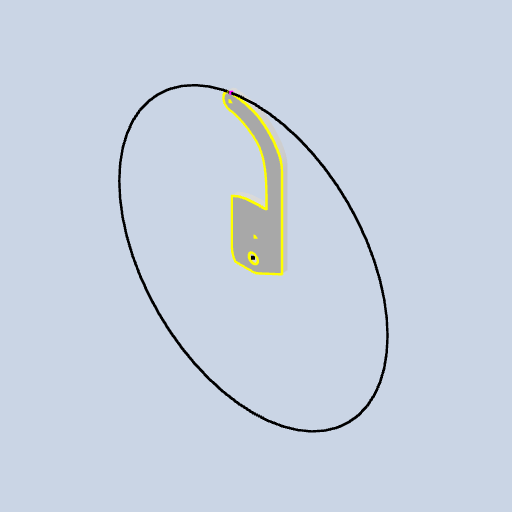
# Autodesk Inventor part: limit_arm
Saved by Autodesk Inventor 2022 (Build 260153000, 153)
## iProperties
Created: 2024-10-15
Part Number: limit_arm
Material: Типовые
Document SubType Name: Modeling
Designer: Andrey
Density: 1 g/cm^3
Appearance: По умолчанию
Author: Andrey
Autodesk Inventor part; units mm, degrees
ref_plane "YZ Plane" through (0, 0, 0) normal (1, 0, 0) x (0, 1, 0)
ref_plane "XZ Plane" through (0, 0, 0) normal (0, 1, 0) x (-1, 0, 0)
ref_plane "XY Plane" through (0, 0, 0) normal (0, 0, 1) x (1, 0, 0)
sketch "Эскиз1" plane through (0, 0, 0) normal (0, 0, 1) x (1, 0, 0)
  line L0 (8.4266, -12.65) -> (-2.5734, -12.65)
  line L1 (-2.5734, -12.65) -> (-2.5734, -47.65)
  line L2 (-2.5734, -47.65) -> (8.4266, -47.65)
  line L3 (8.4266, -47.65) -> (8.4266, -82.9136)
  spline S0 degree 4 poles (2.3773, -93.423) (5.3243, -91.0921) (7.8605, -87.681) (8.4266, -85.6037) (8.4266, -82.9136) knots 0.089011 0.089011 0.089011 0.089011 0.089011 1 1 1 1 1
  spline S1 degree 4 poles (1.3465, -94.1725) (1.6324, -93.9967) (1.8997, -93.813) (2.1479, -93.6217) (2.3773, -93.423) knots 0 0 0 0 0 1 1 1 1 1
  spline S2 degree 4 poles (1.2081, -94.2627) (1.2427, -94.2405) (1.2773, -94.218) (1.3119, -94.1954) (1.3465, -94.1725) knots 0 0 0 0 0 1 1 1 1 1
  spline S3 degree 2 poles (-15.5734, -96.9447) (-3.5967, -97.3511) (1.2081, -94.2627) knots 0 0 0 0.59566 0.59566 0.59566
  line L4 (-125.5734, -96.9447) -> (-15.5734, -96.9447)
  spline S4 degree 2 poles (-125.5734, -96.9447) (-137.55, -97.3511) (-142.3548, -94.2627) knots 0 0 0 0.59566 0.59566 0.59566
  spline S5 degree 4 poles (-142.3548, -94.2627) (-145.6699, -92.132) (-148.8913, -88.0811) (-149.5734, -85.8665) (-149.5734, -82.9136) knots 0 0 0 0 0 1 1 1 1 1
  line L5 (-149.5734, -82.9136) -> (-149.5734, -35.15)
  spline S6 degree 2 poles (-125.5734, 36.6447) (-137.55, 37.0511) (-142.3548, 33.9627) knots 0 0 0 0.59566 0.59566 0.59566
  line L6 (-15.5734, 36.6447) -> (-125.5734, 36.6447)
  spline S7 degree 2 poles (-15.5734, 36.6447) (-3.5967, 37.0511) (1.2081, 33.9627) knots 0 0 0 0.59566 0.59566 0.59566
  spline S8 degree 4 poles (1.2081, 33.9627) (4.5231, 31.832) (7.7445, 27.7811) (8.4266, 25.5665) (8.4266, 22.6136) knots 0 0 0 0 0 1 1 1 1 1
  line L7 (8.4266, 22.6136) -> (8.4266, -12.65)
  line L8 (-10.5734, -92.9447) -> (-10.5734, 32.6447)
  line L9 (-10.5734, 32.6447) -> (-130.5734, 32.6447)
  line L10 (-130.5734, 32.6447) -> (-130.5734, -92.9447)
  line L11 (-130.5734, -92.9447) -> (-10.5734, -92.9447)
  line L12 (5.7794, 10.35) -> (5.7794, -10.35)
  line L13 (-8.4266, 10.35) -> (5.7794, 10.35)
  line L14 (-8.4266, -10.35) -> (-8.4266, 10.35)
  line L15 (5.7794, -10.35) -> (-8.4266, -10.35)
  circle A0 centre (-0.824, -6.35) radius 2.1
  line L16 (-10.5734, 32.6447) -> (-10.5734, -92.9447)
  line L17 (-10.5734, -92.9447) -> (-130.5734, -92.9447)
  line L18 (-130.5734, -92.9447) -> (-130.5734, 32.6447)
  line L19 (-130.5734, 32.6447) -> (-10.5734, 32.6447)
  line L20 (8.4266, -47.65) -> (-2.5734, -47.65)
  line L21 (-2.5734, -47.65) -> (-2.5734, -12.65)
  line L22 (-2.5734, -12.65) -> (8.4266, -12.65)
  line L23 (8.4266, 22.6136) -> (8.4266, -12.65)
  spline S9 degree 4 poles (1.2081, 33.9627) (4.5231, 31.832) (7.7445, 27.7811) (8.4266, 25.5665) (8.4266, 22.6136) knots 0 0 0 0 0 1 1 1 1 1
  spline S10 degree 2 poles (-15.5734, 36.6447) (-3.5967, 37.0511) (1.2081, 33.9627) knots 0 0 0 0.59566 0.59566 0.59566
  line L24 (-125.5734, 36.6447) -> (-15.5734, 36.6447)
  spline S11 degree 2 poles (-142.3548, 33.9627) (-137.55, 37.0511) (-125.5734, 36.6447) knots -0.59566 -0.59566 -0.59566 0 0 0
  spline S12 degree 4 poles (-142.3548, 33.9627) (-145.6699, 31.832) (-148.8913, 27.7811) (-149.5734, 25.5665) (-149.5734, 22.6136) knots 0 0 0 0 0 1 1 1 1 1
  line L25 (-149.5734, 22.6136) -> (-149.5734, -25.15)
  spline S13 degree 2 poles (-125.5734, -96.9447) (-137.55, -97.3511) (-142.3548, -94.2627) knots 0 0 0 0.59566 0.59566 0.59566
  line L26 (-15.5734, -96.9447) -> (-125.5734, -96.9447)
  spline S14 degree 2 poles (-15.5734, -96.9447) (-3.5967, -97.3511) (1.2081, -94.2627) knots 0 0 0 0.59566 0.59566 0.59566
  spline S15 degree 4 poles (1.2081, -94.2627) (1.2427, -94.2405) (1.2773, -94.218) (1.3119, -94.1954) (1.3465, -94.1725) knots 0 0 0 0 0 1 1 1 1 1
  spline S16 degree 4 poles (2.3773, -93.423) (2.1479, -93.6217) (1.8997, -93.813) (1.6324, -93.9967) (1.3465, -94.1725) knots 0 0 0 0 0 1 1 1 1 1
  spline S17 degree 4 poles (2.3773, -93.423) (5.3243, -91.0921) (7.8605, -87.681) (8.4266, -85.6037) (8.4266, -82.9136) knots 0.089011 0.089011 0.089011 0.089011 0.089011 1 1 1 1 1
  line L27 (8.4266, -47.65) -> (8.4266, -82.9136)
  circle A1 centre (-0.824, -6.35) radius 3.8
  line L28 (-0.824, -6.35) -> (0.782, -9.794)
  line L29 (0.782, -9.794) -> (8.4266, -6.2292)
  line L30 (-0.824, -6.35) -> (-0.824, -10.35)
  circle A2 centre (-8.0734, 33.9917) radius 2.5
  line L31 (-8.0734, 33.9917) -> (-7.8457, 36.4813)
  spline S18 degree 4 poles (-8.3011, 31.5021) (-5.572, 31.2525) (-0.0854, 27.7372) (3.5121, 26.3853) (3.4266, 14.7728) (3.4266, 10.35) knots 0 0 0 0 0 0.467272 1 1 1 1 1
  line L32 (8.4266, 10.35) -> (3.4266, 10.35)
  line L33 (-7.8457, 36.4813) -> (-8.3011, 31.5021)
  line L34 (-2.0361, 28.9154) -> (1.2081, 33.9627)
  line L35 (-0.824, -10.15) -> (-7.824, -10.15)
  line L36 (-7.824, -10.15) -> (-7.824, 7.7089)
  line L37 (-7.824, 7.7089) -> (3.4266, 7.7089)
  line L38 (3.4266, 7.7089) -> (3.4266, 10.35)
  line L39 (-8.7741, -6.8356) -> (-1.2266, 9.35)
  line L40 (-8.7741, -6.8356) -> (-2.4299, -9.794)
  line L41 (-1.2266, 9.35) -> (4.6043, 6.631)
  circle A3 centre (-0.824, -6.35) radius 7
  circle A4 centre (-0.824, -6.35) radius 15.7052
  line L42 (-1.2266, 9.35) -> (3.4266, 9.4693)
  circle A5 centre (-0.824, -6.35) radius 1.5
  line L43 (-138.5734, -25.15) -> (-149.5734, -25.15)
  line L44 (-149.5734, -25.15) -> (-149.5734, 22.6136)
  line L45 (-149.5734, -35.15) -> (-138.5734, -35.15)
  line L46 (-138.5734, -35.15) -> (-138.5734, -25.15)
  line L47 (-149.5734, -25.15) -> (-138.5734, -25.15)
  line L48 (-138.5734, -25.15) -> (-138.5734, -35.15)
  line L49 (-138.5734, -35.15) -> (-149.5734, -35.15)
  line L50 (-149.5734, -35.15) -> (-149.5734, -82.9136)
  line L51 (-9.8234, -70.25) -> (-9.8234, -63.25)
  line L52 (-9.8234, -63.25) -> (4.1266, -63.25)
  line L53 (4.1266, -63.25) -> (4.1266, -70.25)
  line L54 (4.1266, -70.25) -> (-9.8234, -70.25)
  line L55 (-9.9734, 2.95) -> (-9.9734, 9.95)
  line L56 (-9.9734, 9.95) -> (4.1266, 9.95)
  line L57 (4.1266, 9.95) -> (4.1266, 2.95)
  line L58 (4.1266, 2.95) -> (-9.9734, 2.95)
  line L59 (-9.8234, -63.25) -> (-9.8234, -70.25)
  line L60 (-9.8234, -70.25) -> (4.1266, -70.25)
  line L61 (4.1266, -70.25) -> (4.1266, -63.25)
  line L62 (4.1266, -63.25) -> (-9.8234, -63.25)
  line L63 (-9.9734, 9.95) -> (-9.9734, 2.95)
  line L64 (-9.9734, 2.95) -> (4.1266, 2.95)
  line L65 (4.1266, 2.95) -> (4.1266, 9.95)
  line L66 (4.1266, 9.95) -> (-9.9734, 9.95)
  spline S19 degree 4 poles (-142.3548, -94.2627) (-145.6699, -92.132) (-148.8913, -88.0811) (-149.5734, -85.8665) (-149.5734, -82.9136) knots 0 0 0 0 0 1 1 1 1 1
  spline S20 degree 4 poles (-142.3548, 33.9627) (-145.6699, 31.832) (-148.8913, 27.7811) (-149.5734, 25.5665) (-149.5734, 22.6136) knots 0 0 0 0 0 1 1 1 1 1
  point P0 (0, 0)
  point P1 (1.9242, 24.3867)
  point P2 (3.4266, 9.35)
  point P3 (-6.5685, -10.35)
  point P4 (5.7794, -8.6727)
  point P5 (6.11, -7.3095)
  point P6 (-7.886, 36.4854)
  point P7 (-7.824, -6.35)
  point P8 (-6.7027, -10.15)
  point P9 (-7.8466, 36.4837)
  point P10 (1.2103, 33.9674)
  point P11 (-7.8461, 36.4827)
  point P12 (1.2099, 33.9666)
  point P13 (-7.8465, 36.4834)
  point P14 (-7.8062, 36.4797)
  point P15 (1.2097, 33.9661)
  point P16 (-7.8463, 36.4828)
  point P17 (-7.8061, 36.4794)
  point P18 (1.2094, 33.9656)
  point P19 (-7.8462, 36.4824)
  point P20 (-7.846, 36.4824)
  point P21 (-7.8462, 36.4824)
  point P22 (1.2092, 33.9651)
  point P23 (-7.8457, 36.4813)
  point P24 (1.2089, 33.9645)
  point P25 (-7.8461, 36.4821)
  point P26 (-7.8058, 36.4784)
  point P27 (1.2087, 33.964)
  point P28 (-7.8458, 36.4813)
  point P29 (-7.8057, 36.4781)
  point P30 (1.2085, 33.9635)
  point P31 (-7.8458, 36.4813)
  point P32 (-7.8457, 36.4813)
  dimension "d0" = 7.6
  dimension "d1" = 25
  dimension "d2" = 5
  dimension "d3" = 5
  dimension "d4" = 6
  dimension "d6" = 7
  dimension "d7" = 25
  dimension "d8" = 7
  dimension "d9" = 1
  dimension "d13" = 3
  constraints: 30 end point, 8 perpendicular, 7 point on circle, 7 point on line, 5 centre point, 5 tangent, 4 coincident, 1 collinear, 1 horizontal, 8 other
  measures "d0" diameter of A1
  measures "d1" angle of L30 L28
  measures "d2" diameter of A2
  measures "d3" distance of L32.start L32.end
  measures "d4" distance of L34.end L34.start
  measures "d6" distance of L35.start L35.end
  measures "d7" angle of L39 L36
  measures "d8" distance of L39.start L40.end
  measures "d9" distance from line of L39.end L13
  measures "d13" diameter of A5
extrude "Выдавливание1" add sketch "Эскиз1" along normal blind 2 contours L29 A3 L12 A4 L7 | A4 L12 L32 L7 | L29 L12 A3 | L32 L13 S18 L34 S8 L7 | A4 L57 L56 L38 L13 L12 | L12 A3 L39 L58 L57 A4 | L29 A1 L40 A3 L12 | A3 L40 A1 L35 | L30 A0 L28 A1 | A1 L28 A0 L30 | L57 L41 L37 L38 A4 | A4 L38 L56 L57 | L30 A5 L28 A0 | A0 L28 A5 L30 | L34 S18 A2 S7 | A3 L36 L39 | L39 L36 L58 | A4 L42 L38 | L38 L37 L41 A4 | L57 L58 L39 L37 L41 | L31 L33 A2 | A2 L33 L31 | L58 L36 L37 L39 | L41 L37 L39 | L39 L37 A4 picked at (5.8525, -5.4253)
sketch "Эскиз2" plane through (0, 0, 2) normal (0, 0, 1) x (1, 0, 0)
  line L0 (8.4266, -6.2292) -> (8.4266, 22.6136) projected
  line L1 (0.782, -9.794) -> (8.4266, -6.2292) projected
  arc A0 (-0.824, -10.15) -> (0.782, -9.794) centre (-0.824, -6.35) ccw projected
  line L2 (-6.7027, -10.15) -> (-0.824, -10.15) projected
  arc A1 (-7.824, -6.35) -> (-6.7027, -10.15) centre (-0.824, -6.35) ccw projected
  line L3 (-7.824, 7.7089) -> (-7.824, -6.35) projected
  arc A2 (-1.2266, 9.35) -> (-7.824, 7.7089) centre (-0.824, -6.35) ccw projected
  line L4 (3.4266, 9.4693) -> (-1.2266, 9.35) projected
  line L5 (3.4266, 10.35) -> (3.4266, 9.4693) projected
  arc A3 (-7.8457, 36.4813) -> (-8.3011, 31.5021) centre (-8.0734, 33.9917) ccw projected
  circle A4 centre (-0.824, -6.35) radius 1.5 projected
  circle A5 centre (-0.824, -6.35) radius 43.4879
  arc A6 (-7.8458, 36.4818) -> (-8.3011, 31.5021) centre (-8.0734, 33.9917) ccw projected
  point P0 (0, 0)
  point P1 (-7.8466, 36.4842)
  point P2 (-7.8463, 36.4831)
  constraints: 1 centre point, 1 coincident, 6 other
